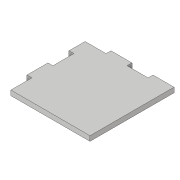
# Autodesk Inventor part: base
Saved by Autodesk Inventor 2017 (Build 210142000, 142)
## iProperties
Created: 2019-05-21
Part Number: base
Material: Generic
Document SubType Name: Modeling
Designer: markg
Density: 1 g/cm^3
Appearance: Default
Author: markg
Autodesk Inventor part; units mm, degrees
ref_plane "YZ Plane" through (0, 0, 0) normal (1, 0, 0) x (0, 1, 0)
ref_plane "XZ Plane" through (0, 0, 0) normal (0, 1, 0) x (-1, 0, 0)
ref_plane "XY Plane" through (0, 0, 0) normal (0, 0, 1) x (1, 0, 0)
sketch "Sketch1" plane through (0, 0, 0) normal (0, 1, 0) x (-1, 0, 0)
  line L0 (-25.4, 25.4) -> (25.4, 25.4)
  line L1 (25.4, 25.4) -> (25.4, -25.4)
  line L2 (25.4, -25.4) -> (-25.4, -25.4)
  line L3 (-25.4, -25.4) -> (-25.4, 25.4)
  line L4 (-25.4, 25.4) -> (25.4, -25.4) construction
  line L5 (25.4, 25.4) -> (-25.4, -25.4) construction
  point P0 (0, 0)
  dimension "d0" = 50.8
  dimension "d1" = 50.8
  constraints: 12 end point, 2 midpoint, 2 parallel, 1 horizontal, 1 perpendicular
  measures "d0" distance of L1.end L2.end
  measures "d1" distance of L0.end L1.end
extrude "Extrusion1" add sketch "Sketch1" along normal blind 2.9718
sketch "Sketch2" plane through (0, 2.9718, 0) normal (0, 1, 0) x (1, 0, 0)
  line L0 (-25.4, -25.4) -> (25.4, -25.4) projected
  line L1 (-25.4, -25.4) -> (-22.4282, -25.4)
  line L2 (-22.4282, -25.4) -> (-22.4282, -12.7)
  line L3 (-22.4282, -12.7) -> (-25.4, -12.7)
  line L4 (-25.4, -12.7) -> (-25.4, -25.4)
  line L5 (-25.4, 25.4) -> (-25.4, -25.4) projected
  line L6 (-25.4, 0) -> (-22.4282, 0)
  line L7 (-22.4282, 0) -> (-22.4282, 12.7)
  line L8 (-22.4282, 12.7) -> (-25.4, 12.7)
  line L9 (-25.4, 12.7) -> (-25.4, 0)
  line L10 (-25.4, 25.4) -> (-12.7, 25.4)
  line L11 (-12.7, 25.4) -> (-12.7, 22.4282)
  line L12 (-12.7, 22.4282) -> (-25.4, 22.4282)
  line L13 (-25.4, 22.4282) -> (-25.4, 25.4)
  line L14 (25.4, 25.4) -> (-25.4, 25.4) projected
  line L15 (0, 25.4) -> (12.7, 25.4)
  line L16 (12.7, 25.4) -> (12.7, 22.4282)
  line L17 (12.7, 22.4282) -> (0, 22.4282)
  line L18 (0, 22.4282) -> (0, 25.4)
  point P0 (0, 0)
  dimension "d4" = 2.9718
  dimension "d5" = 12.7
  dimension "d6" = 2.9718
  dimension "d7" = 12.7
  dimension "d8" = 12.7
  dimension "d9" = 2.9718
  dimension "d10" = 12.7
  dimension "d11" = 2.9718
  constraints: 32 end point, 8 parallel, 4 horizontal, 4 perpendicular, 2 midpoint
  measures "d4" distance of L3.end L2.end
  measures "d5" distance of L2.end L1.end
  measures "d6" distance of L8.end L7.end
  measures "d7" distance of L7.end L6.end
  measures "d8" distance of L11.end L12.end
  measures "d9" distance of L10.end L11.end
  measures "d10" distance of L16.end L17.end
  measures "d11" distance of L15.end L16.end
extrude "Extrusion2" cut sketch "Sketch2" against normal blind 2.9718
body "Solid1"
